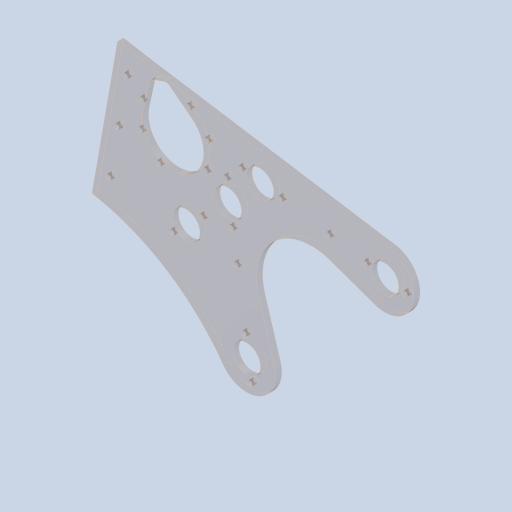
# Autodesk Inventor part: GP9-002
Saved by Autodesk Inventor 2023.4 (Build 274418000, 418)
## iProperties
Created: 2025-02-24
Part Number: GP9-002
Material: Polycarbonate, Smoke
Document SubType Name: Modeling
Designer: dlangdon
Density: 1.2 g/cm^3
Appearance: Polycarbonate - Smoked
Author: dlangdon
Autodesk Inventor part; units mm, degrees
ref_plane "YZ Plane" through (0, 0, 0) normal (1, 0, 0) x (0, 1, 0)
ref_plane "XZ Plane" through (0, 0, 0) normal (0, 1, 0) x (-1, 0, 0)
ref_plane "XY Plane" through (0, 0, 0) normal (0, 0, 1) x (1, 0, 0)
sketch "Sketch1" plane through (0, 0, 0) normal (0, 0, 1) x (1, 0, 0)
  circle A0 centre (71.842, 71.842) radius 50.8 construction
  circle A1 centre (-71.842, -71.842) radius 50.8 construction
  circle A2 centre (0, 0) radius 50.8 construction
  line L0 (-35.921, -35.921) -> (35.921, 35.921) construction
  line L1 (71.842, 71.842) -> (-71.842, -71.842) construction
  line L2 (-4.3707, 6.2419) -> (-4.3707, 50.6116) construction
  line L3 (-226.8798, -122.642) -> (638.5123, -122.642) construction
  circle A3 centre (147.8406, -65.492) radius 57.15 construction
  circle A4 centre (71.842, 71.842) radius 14.2875
  circle A5 centre (-71.842, -71.842) radius 14.2875
  circle A6 centre (-4.3707, 6.2419) radius 57.15 construction
  circle A7 centre (-71.842, -71.842) radius 30.1625 construction
  circle A8 centre (71.842, 71.842) radius 30.1625 construction
  circle A9 centre (-58.1541, 92.3085) radius 14.2875
  line L4 (-58.1541, 92.3085) -> (71.842, 71.842) construction
  circle A10 centre (71.842, 71.842) radius 14.3256 construction
  circle A11 centre (-71.842, -71.842) radius 14.3256 construction
  circle A12 centre (-91.5234, 58.2753) radius 14.2875
  line L5 (-71.842, -71.842) -> (-91.5234, 58.2753) construction
  circle A13 centre (-91.5234, 58.2753) radius 23.8316 construction
  circle A14 centre (-58.1541, 92.3085) radius 23.8316 construction
  line L6 (14.744, 60.1006) -> (61.7538, 43.4167)
  line L7 (-42.9911, -63.0445) -> (-59.0357, -10.4271)
  arc A15 (14.744, 60.1006) -> (-59.0357, -10.4271) centre (-4.3707, 6.2419) ccw
  line L8 (-206.2644, 146.6716) -> (-181.2503, 142.2609)
  line L9 (-181.2503, 142.2609) -> (-207.7142, -7.8238) construction
  line L10 (-207.7142, -7.8238) -> (-232.7284, -3.4132) construction
  line L11 (-232.7284, -3.4132) -> (-206.2644, 146.6716) construction
  line L12 (-248.4004, -92.2937) -> (35.0702, -142.2772) construction
  line L13 (-201.8537, 171.6857) -> (174.1389, 105.388) construction
  line L14 (-201.8537, 171.6857) -> (-248.4004, -92.2937) construction
  circle A16 centre (-148.3894, 90.9308) radius 31.75
  line L15 (-87.9592, 34.7118) -> (-79.4396, -21.6134) construction
  circle A17 centre (12.2511, 81.224) radius 9.525 construction
  line L16 (-193.7573, 144.4662) -> (-220.2213, -5.6185) construction
  line L17 (-198.168, 119.4521) -> (-215.8106, 19.3956) construction
  circle A18 centre (-148.3894, 90.9308) radius 17.4625 construction
  circle A19 centre (-148.3894, 90.9308) radius 9.525
  circle A20 centre (-58.1541, 92.3085) radius 30.1816 construction
  line L18 (-206.2644, 146.6716) -> (-232.7284, -3.4132)
  arc A21 (61.7538, 43.4167) -> (76.5373, 101.6369) centre (71.842, 71.842) ccw
  arc A22 (-96.3859, -89.3742) -> (-42.9911, -63.0445) centre (-71.842, -71.842) ccw
  line L19 (-148.3894, 90.9308) -> (-131.98, 96.9034) construction
  line L20 (-114.0789, 103.4189) -> (-182.6999, 78.4428) construction
  circle A23 centre (-182.6999, 78.4428) radius 4.7625 construction
  line L21 (0, 0) -> (-4.3707, 6.2419) construction
  circle A24 centre (71.842, 71.842) radius 28.6512 construction
  line L22 (64.3236, 44.1949) -> (-61.9034, 78.5217) construction
  line L23 (73.1822, 100.4619) -> (-57.4858, 106.5804) construction
  line L24 (-181.2503, 142.2609) -> (76.5373, 101.6369)
  line L25 (-148.3894, 90.9308) -> (-134.7483, 17.1109) construction
  circle A25 centre (-134.7483, 17.1109) radius 31.75 construction
  circle A26 centre (-134.7483, 17.1109) radius 14.2875
  line L26 (-91.5234, 58.2753) -> (-134.7483, 17.1109) construction
  circle A27 centre (-148.3894, 90.9308) radius 25.4 construction
  arc A28 (-96.3859, -89.3742) -> (-232.7284, -3.4132) centre (-269.7173, -213.1878) ccw
  circle A29 centre (-148.3894, 90.9308) radius 36.5125 construction
  line L27 (-181.481, 106.3617) -> (-148.3894, 90.9308) construction
  point P0 (-83.6994, 6.5492)
  point P1 (-206.9893, 69.4239)
  point P2 (-206.9893, 69.4239)
  point P3 (-145.3571, 108.1281)
  point P4 (-161.7664, 102.1555)
  point P5 (-164.7988, 84.9583)
  point P6 (-151.4217, 73.7336)
  point P7 (-135.0123, 79.7062)
  point P8 (-124.5212, 99.6182)
  point P9 (-143.9787, 115.945)
  point P10 (-167.8469, 107.2576)
  point P11 (-172.2576, 82.2435)
  point P12 (-152.8001, 65.9167)
  point P13 (-128.9319, 74.604)
  point P14 (-160.8774, 125.2414)
  point P15 (-182.6999, 78.4428)
  point P16 (-135.9014, 56.6203)
  point P17 (-132.9585, 124.0224)
  point P18 (-163.8202, 57.8393)
  point P19 (-115.2978, 75.5)
  dimension "d7" = 101.6
  dimension "d18" = 47.6631
  dimension "d34" = 34.925
  dimension "d65" = 50.8
  dimension "d3" = 45
  dimension "d4" = 0
  dimension "d8" = 101.6
  dimension "d9" = 28.575
  dimension "d10" = 101.6
  dimension "d11" = 114.3
  dimension "d12" = 114.3
  dimension "d13" = 15.875
  dimension "d14" = 15.875
  dimension "d15" = 131.5974
  dimension "d16" = 28.6512
  dimension "d17" = 131.5974
  dimension "d19" = 47.6631
  dimension "d22" = 25.4
  dimension "d23" = 152.4
  dimension "d26" = 268.0517
  dimension "d27" = 63.5
  dimension "d30" = 203.2
  dimension "d31" = 10
  dimension "d32" = 19.05
  dimension "d33" = 101.6
  dimension "d35" = 19.05
  dimension "d36" = 6.35
  dimension "d40" = 360
  dimension "d44" = 9.525
  dimension "d55" = 80
  dimension "d56" = 7.62
  dimension "d57" = 25.4
  dimension "d58" = 57.3024
  dimension "d59" = 63.5
  dimension "d60" = 75.0697
  dimension "d61" = 59.69
  dimension "d62" = 55
  dimension "d68" = 360
  dimension "d70" = 41.275
  dimension "d71" = 60
  dimension "d88" = 360
  dimension "d93" = 360
  dimension "d95" = 45
  constraints: 56 end point, 26 centre point, 24 coincident, 23 point on circle, 16 tangent, 7 midpoint, 6 equal radius, 5 point on line, 4 collinear, 4 parallel, 2 horizontal, 1 concentric, 1 perpendicular, 1 vertical, 39 other
  measures "d3" angle of L2 L0
  measures "d4" distance between parallel lines of L0 L1
  measures "d8" diameter of A2
  measures "d9" diameter of A4
  measures "d10" diameter of A0
  measures "d11" diameter of A3
  measures "d12" diameter of A6
  measures "d13" radial gap between concentric circles of A5 A7
  measures "d14" radial gap between concentric circles of A4 A8
  measures "d15" distance of L4.start L4.end
  measures "d16" diameter of A10
  measures "d17" distance of L5.start L5.end
  measures "d19" diameter of A14
  measures "d22" distance of L9.end L10.end
  measures "d23" distance of L10.end L8.start
  measures "d26" distance of L13.start L12.start
  measures "d27" diameter of A16
  measures "d30" distance from line of point (0, 0) L9
  measures "d31" angle of L3 L12
  measures "d32" diameter of A17
  measures "d33" distance of L17.start L17.end
  measures "d35" diameter of A19
  measures "d36" radial gap between concentric circles of A14 A20
  measures "d44" diameter of A23
  measures "d55" angle of L1 L21
  measures "d56" distance of L21.start L21.end
  measures "d57" distance between parallel lines of L13 L8
  measures "d58" diameter of A24
  measures "d59" diameter of A25
  measures "d60" distance of L19.start L25.end
  measures "d61" distance of L26.start L26.end
  measures "d62" angle of L15 L26
  measures "d70" distance from line of L9 L19.start
  measures "d71" angle of L9 L20
  measures "d95" angle of L20 L27
extrude "Extrusion1" add sketch "Sketch1" along normal blind 6.35 contours A15 L7 A22 A28 L18 L8 L24 A21 L6
hole "Hole1" at (12.2511, 81.224, 0) at (-198.168, 119.4521, 0) at (-206.9893, 69.4239, 0) at (-215.8106, 19.3956, 0) at (-131.98, 96.9034, 0) at (-145.3571, 108.1281, 0) at (-161.7664, 102.1555, 0) at (-164.7988, 84.9583, 0) at (-151.4217, 73.7336, 0) at (-135.0123, 79.7062, 0) at (-152.8001, 65.9167, 0) at (-172.2576, 82.2435, 0) at (-167.8469, 107.2576, 0) at (-143.9787, 115.945, 0) at (-124.5212, 99.6182, 0) at (-128.9319, 74.604, 0) at (-83.6994, 6.5492, 0) at (-132.9585, 124.0224, 0) at (-181.481, 106.3617, 0) at (-163.8202, 57.8393, 0) at (-115.2978, 75.5, 0) at (-182.6999, 78.4428, 0) at (-114.0789, 103.4189, 0) direction (0, 0, 1) diameter 5.1054 end through all clearance for "Flat Head Machine Screw (82)" size "#10" standard "Ansi Unified Screw Threads"
sketch "Sketch2" plane through (0, 0, 6.35) normal (0, 0, 1) x (1, 0, 0)
  circle A0 centre (-215.8106, 19.3956) radius 2.5527 construction
  circle A1 centre (-198.168, 119.4521) radius 2.5527 construction
  circle A2 centre (12.2511, 81.224) radius 2.5527 construction
  circle A3 centre (-206.9893, 69.4239) radius 2.5527 construction
  circle A4 centre (-83.6994, 6.5492) radius 2.5527 construction
  line L0 (-42.9911, -63.0445) -> (-59.0357, -10.4271) construction
  arc A5 (14.744, 60.1006) -> (-59.0357, -10.4271) centre (-4.3707, 6.2419) ccw construction
  line L1 (14.744, 60.1006) -> (61.7538, 43.4167) construction
  arc A6 (61.7538, 43.4167) -> (76.5373, 101.6369) centre (71.842, 71.842) ccw construction
  line L2 (76.5373, 101.6369) -> (-181.2503, 142.2609) construction
  line L3 (-181.2503, 142.2609) -> (-206.2644, 146.6716) construction
  line L4 (-206.2644, 146.6716) -> (-232.7284, -3.4132) construction
  arc A7 (-96.3859, -89.3742) -> (-232.7284, -3.4132) centre (-269.7173, -213.1878) ccw construction
  arc A8 (-96.3859, -89.3742) -> (-42.9911, -63.0445) centre (-71.842, -71.842) ccw construction
  circle A9 centre (-91.5234, 58.2753) radius 14.2875 construction
  circle A10 centre (-134.7483, 17.1109) radius 14.2875 construction
  circle A11 centre (-58.1541, 92.3085) radius 14.2875 construction
  circle A12 centre (-71.842, -71.842) radius 14.2875 construction
  circle A13 centre (71.842, 71.842) radius 14.2875 construction
  line L5 (-74.9855, -51.0599) -> (-68.6986, -92.6242) construction
  line L6 (-149.969, 2.6158) -> (-119.5276, 31.606) construction
  line L7 (-94.6669, 79.0574) -> (-88.3799, 37.4932) construction
  line L8 (-78.9169, 95.5774) -> (-37.3914, 89.0396) construction
  line L9 (51.0793, 75.1109) -> (92.6048, 68.5732) construction
  circle A14 centre (-91.5234, 58.2753) radius 14.2875 construction
  line L10 (-58.1541, 92.3085) -> (-91.5234, 58.2753) construction
  line L11 (-58.1541, 92.3085) -> (71.842, 71.842) construction
  line L12 (-91.5234, 58.2753) -> (-134.7483, 17.1109) construction
  line L13 (-91.5234, 58.2753) -> (-71.842, -71.842) construction
  point P0 (0, 0)
  dimension "d72" = 42.037
  constraints: 19 end point, 14 coincident, 5 collinear, 5 midpoint, 4 equal length
  measures "d72" distance of L5.start L5.end
hole "Hole2" at (-74.9855, -51.0599, 6.35) at (-119.5276, 31.606, 6.35) at (-68.6986, -92.6242, 6.35) at (-149.969, 2.6158, 6.35) at (-88.3799, 37.4932, 6.35) at (-94.6669, 79.0574, 6.35) at (-37.3914, 89.0396, 6.35) at (-78.9169, 95.5774, 6.35) at (92.6048, 68.5732, 6.35) at (51.0793, 75.1109, 6.35) direction (0, 0, -1) diameter 5.1054 end through all clearance for "Flat Head Machine Screw (82)" size "#10" standard "Ansi Unified Screw Threads"
sketch "Sketch3" plane through (0, 0, 6.35) normal (0, 0, 1) x (1, 0, 0)
  circle A0 centre (-148.3894, 90.9308) radius 31.75 projected
  line L0 (-179.4216, 97.6439) -> (-172.5428, 129.4424)
  line L1 (-172.5428, 129.4424) -> (-154.6416, 135.9579)
  line L2 (-154.6416, 135.9579) -> (-128.9324, 116.0205)
  circle A1 centre (-114.0789, 103.4189) radius 2.5527 projected
  circle A2 centre (-183.1052, 76.1445) radius 2.5527 projected
  line L3 (-113.3876, 101.5196) -> (-183.1052, 76.1445) construction
  line L4 (-183.1052, 76.1445) -> (-147.6981, 89.0316)
  line L5 (-148.3894, 90.9308) -> (-163.5922, 132.7002) construction
  point P0 (0, 0)
  dimension "d80" = 44.45
  dimension "d82" = 19.05
  constraints: 12 end point, 2 point on circle, 2 tangent, 1 collinear, 1 equal length, 1 midpoint, 1 perpendicular
  measures "d80" distance from line of L4.end L1
  measures "d82" distance of L0.end L1.end
extrude "Extrusion2" cut sketch "Sketch3" against normal through all contours A0 L0 L1 L2
fillet "Fillet1" radius 6.35 2 edges at (-172.5428, 129.4424, 3.175) (-154.6416, 135.9579, 3.175)
body "Solid1"
